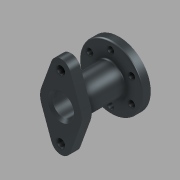
# Autodesk Inventor part: Lab6A01209499P1
Saved by Autodesk Inventor 2020 (Build 240168000, 168)
## iProperties
Created: 2019-09-20
Part Number: Lab6A01209499P1
Material: Hierro, fundido
Document SubType Name: Modeling
Designer: gerar
Density: 7.15 g/cm^3
Appearance: Gris hierro
Author: gerar
Autodesk Inventor part; units mm, degrees
ref_plane "YZ Plane" through (0, 0, 0) normal (1, 0, 0) x (0, 1, 0)
ref_plane "XZ Plane" through (0, 0, 0) normal (0, 1, 0) x (-1, 0, 0)
ref_plane "XY Plane" through (0, 0, 0) normal (0, 0, 1) x (1, 0, 0)
sketch "Boceto1" plane through (0, 0, 0) normal (1, 0, 0) x (0, 1, 0)
  line L0 (10, -25) -> (10, -70)
  line L1 (10, -70) -> (38, -70)
  line L2 (38, -70) -> (38, -60)
  line L3 (38, -60) -> (18, -60)
  line L4 (18, -60) -> (18, 0)
  line L5 (18, 0) -> (13, 0)
  line L6 (-7.6, 0) -> (45.6, 0) construction
  line L7 (0, -84) -> (0, 14) projected
  line L8 (13, 0) -> (13, -25)
  line L9 (13, -25) -> (10, -25)
  point P0 (0, 0)
  dimension "d6" = 20
  dimension "d8" = 36
  dimension "d9" = 10
  dimension "d10" = 76
  dimension "d11" = 26
  dimension "d12" = 25
  dimension "d35" = 70
  constraints: 16 end point, 6 perpendicular, 2 vertical, 1 horizontal, 2 other
  measures "d6" diameter of L0 L7
  measures "d8" diameter of L4 L7
  measures "d9" distance between parallel lines of L1 L3
  measures "d10" diameter of L2 L7
  measures "d11" diameter of L8 L7
  measures "d12" distance of L5.end L8.end
  measures "d35" distance between parallel lines of L5 L1
revolve "Revolución1" add sketch "Boceto1" angle 360 about axis through (0, 0, -10) along (0, 0, 1)
sketch "Boceto2" plane through (0, 0, 0) normal (0, 0, 1) x (1, 0, 0)
  line L0 (-53.2, 0) -> (53.2, 0) construction
  line L1 (0, -70) -> (0, 70) construction
  arc A0 (11.2759, 42.1053) -> (-11.2759, 42.1053) centre (0, 38) ccw
  line L2 (-11.2759, 42.1053) -> (-23.4915, 8.5526)
  line L3 (11.2759, 42.1053) -> (23.4915, 8.5526)
  arc A1 (-23.4915, 8.5526) -> (-25, 0) centre (0, 0) ccw
  arc A2 (25, 0) -> (23.4915, 8.5526) centre (0, 0) ccw
  circle A3 centre (0, 38) radius 5
  arc A4 (-11.2759, -42.1053) -> (11.2759, -42.1053) centre (0, -38) ccw
  line L4 (-11.2759, -42.1053) -> (-23.4915, -8.5526)
  line L5 (11.2759, -42.1053) -> (23.4915, -8.5526)
  arc A5 (-25, 0) -> (-23.4915, -8.5526) centre (0, 0) ccw
  arc A6 (23.4915, -8.5526) -> (25, 0) centre (0, 0) ccw
  circle A7 centre (0, -38) radius 5
  circle A8 centre (0, 0) radius 13
  dimension "d14" = 12
  dimension "d15" = 25
  dimension "d16" = 38
  dimension "d17" = 10
  constraints: 12 point on circle, 9 centre point, 8 end point, 6 symmetric about line, 4 coincident, 4 tangent, 3 point on line, 1 concentric, 4 other
  measures "d14" radius of A0
  measures "d15" radius of A2
  measures "d16" distance of point (0, 0) A0.centre
  measures "d17" diameter of A3
extrude "Extrusión1" add sketch "Boceto2" against normal blind 12
sketch "Boceto3" plane through (0, 0, -70) normal (0, 0, -1) x (-1, 0, 0)
  circle A0 centre (0, 0) radius 29 construction
  point P0 (0, 29)
  dimension "d20" = 58
  constraints: 1 coincident, 1 vertical alignment, 2 other
hole "Agujero1" at (0, 29, -70) direction (0, 0, 1) diameter 8 depth 10
pattern_circular "Patrón circular1" count 6 over 360 about axis through (0, 0, -10) along (0, 0, 1) of "Agujero1"
chamfer "Chaflán1" distance 3 angle 45 1 edges at (0, -13, 0) measured on face at (11.9516, -17.6559, 0)
fillet "Empalme1" radius 2 2 edges at (0, -18, -60) (0, -38, -60)
